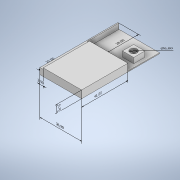
# Autodesk Inventor part: support_1
Saved by Autodesk Inventor 2020 (Build 240168000, 168)
## iProperties
Created: 2019-11-28
Part Number: support_1
Material: Generic
Document SubType Name: Modeling
Designer: sl65b
Density: 1 g/cm^3
Appearance: Default
Author: sl65b
Autodesk Inventor part; units mm, degrees
ref_plane "YZ Plane" through (0, 0, 0) normal (1, 0, 0) x (0, 1, 0)
ref_plane "XZ Plane" through (0, 0, 0) normal (0, 1, 0) x (-1, 0, 0)
ref_plane "XY Plane" through (0, 0, 0) normal (0, 0, 1) x (1, 0, 0)
sketch "Sketch1" plane through (0, 0, 0) normal (0, 1, 0) x (-1, 0, 0)
  line L0 (19.325, 34.5) -> (-19.325, 34.5)
  line L1 (-19.325, 34.5) -> (-19.325, -34.5)
  line L2 (-19.325, -34.5) -> (19.325, -34.5)
  line L3 (19.325, -34.5) -> (19.325, 34.5)
  line L4 (19.325, 34.5) -> (-19.325, -34.5) construction
  line L5 (-19.325, 34.5) -> (19.325, -34.5) construction
  point P0 (0, 0)
  dimension "d0" = 38.65
  dimension "d1" = 69
  constraints: 12 end point, 2 midpoint, 2 parallel, 1 horizontal, 1 perpendicular
  measures "d0" distance of L0.start L0.end
  measures "d1" distance of L0.end L1.end
extrude "Extrusion1" add sketch "Sketch1" along normal blind 5.5
sketch "Sketch3" plane through (0, 5.5, 0) normal (0, 1, 0) x (1, 0, 0)
  line L0 (19.325, -34.5) -> (19.325, 34.5) projected
  line L1 (19.325, -34.5) -> (-14.675, -34.5)
  line L2 (-14.675, -34.5) -> (-14.675, 6.5)
  line L3 (-14.675, 6.5) -> (19.325, 6.5)
  line L4 (19.325, 6.5) -> (19.325, -34.5)
  point P0 (0, 0)
  dimension "d4" = 34
  dimension "d5" = 41
  constraints: 8 end point, 2 parallel, 1 horizontal, 1 perpendicular
  measures "d4" distance of L2.end L3.end
  measures "d5" distance of L1.end L2.end
extrude "Extrusion2" add sketch "Sketch3" along normal blind 1.2
sketch "Sketch4" plane through (-19.325, 0, -34.5) normal (-1, 0, 0) x (0, 0, 1)
  point P0 (34.5, 0)
sketch "Sketch5" plane through (0, 5.5, 0) normal (0, 1, 0) x (1, 0, 0)
  line L0 (19.325, 34.5) -> (-19.325, 34.5) projected
  line L1 (19.325, 34.5) -> (11.265, 34.5)
  circle A0 centre (11.265, 19.65) radius 2.4036
  line L2 (-14.675, -34.5) -> (19.325, -34.5) projected
  point P0 (0, 0)
  dimension "d20" = 8.06
  dimension "d21" = 54.15
  constraints: 2 end point, 1 centre point, 1 point on line
  measures "d20" distance of L0.start L1.end
  measures "d21" distance from line of L2 A0.centre
hole "Hole1" at (11.265, 5.5, -19.65) direction (0, -1, 0) diameter 3.5 depth 10.5 tip angle 118 counterbore diameter 6 counterbore depth 2.3
sketch "Sketch6" plane through (0, 5.5, 0) normal (0, 1, 0) x (1, 0, 0)
  line L0 (19.325, -34.5) -> (19.325, 34.5) projected
  line L1 (19.325, 34.5) -> (-16.5957, 34.5)
  line L2 (-16.5957, 34.5) -> (-16.5957, 6.5)
  line L3 (-16.5957, 6.5) -> (19.325, 6.5)
  line L4 (19.325, 6.5) -> (19.325, 34.5)
  line L5 (16.265, 24.65) -> (6.265, 24.65)
  line L6 (6.265, 24.65) -> (6.265, 14.65)
  line L7 (6.265, 14.65) -> (16.265, 14.65)
  line L8 (16.265, 14.65) -> (16.265, 24.65)
  circle A0 centre (11.265, 19.65) radius 1.75 projected
  line L9 (16.265, 24.65) -> (6.265, 14.65) construction
  line L10 (6.265, 24.65) -> (16.265, 14.65) construction
  point P0 (0, 0)
  point P1 (19.325, 6.5)
  dimension "d32" = 10
  dimension "d33" = 10
  dimension "d37" = 28
  constraints: 20 end point, 4 parallel, 2 horizontal, 2 midpoint, 2 perpendicular
  measures "d32" distance of L7.end L6.end
  measures "d33" distance of L6.end L5.end
  measures "d37" distance of L1.end L2.end
extrude "Extrusion3" cut sketch "Sketch6" against normal blind 4.75 contours L3 L2 L1 L0
sketch "Sketch7" plane through (0, 0, 0) normal (0, -1, 0) x (1, 0, 0)
  line L0 (-13.5462, 6.5334) -> (16.4538, 6.5334)
  line L1 (16.4538, 6.5334) -> (16.4538, 31.5334)
  line L2 (16.4538, 31.5334) -> (-13.5462, 31.5334)
  line L3 (-13.5462, 31.5334) -> (-13.5462, 6.5334)
  line L4 (-13.5462, 6.5334) -> (16.4538, 31.5334) construction
  line L5 (16.4538, 6.5334) -> (-13.5462, 31.5334) construction
  point P0 (0, 0)
  point P1 (1.4538, 19.0334)
  dimension "d40" = 30
  dimension "d41" = 25
  constraints: 12 end point, 2 midpoint, 2 parallel, 1 horizontal, 1 perpendicular
  measures "d40" distance of L1.end L2.end
  measures "d41" distance of L0.end L1.end
extrude "Extrusion4" cut sketch "Sketch7" against normal blind 5.75
sketch "Sketch8" plane through (-19.325, 0, -34.5) normal (-1, 0, 0) x (0, 0, 1)
  line L0 (0, 0) -> (69, 0) projected
  line L1 (69, 0) -> (69, 5.5) projected
  line L2 (0, 0) -> (69, 0)
  line L3 (69, 0) -> (69, 5.5)
  line L4 (69, 5.5) -> (0, 5.5)
  line L5 (0, 5.5) -> (0, 0)
  point P0 (34.5, 0)
  constraints: 8 end point, 2 parallel, 1 horizontal, 1 perpendicular
extrude "Extrusion5" cut sketch "Sketch8" against normal blind 1.75
body "Solid1"
